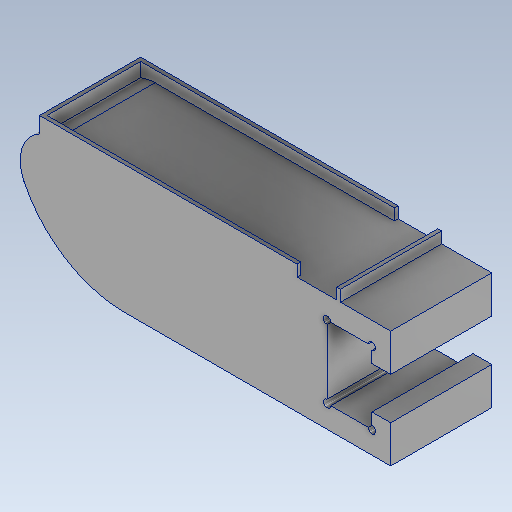
# Autodesk Inventor part: Finray_9_Kerbe_10deg_anschluss_erweitert_9_75 Nut
Saved by Autodesk Inventor 2025.2 (Build 292293000, 293)
## iProperties
Created: 2022-02-28
Part Number: Finray_9_Kerbe_10deg_anschluss_erweitert_9_75 Nut
Material: Generic
Document SubType Name: Modeling
Designer: richa
Density: 1 g/cm^3
Appearance: Aluminum - Flat
Author: richa
## iProperties of the stored document Maria_Greifer_3D-Druck.ipt
Created: 2024-11-10
Part Number: Maria_Greifer_3D-Druck
Material: Generisch
Document SubType Name: Modeling
Designer: maria
Density: 1 g/cm^3
Appearance: Vorgabe
Author: maria
Autodesk Inventor part; units mm, degrees
ref_plane "YZ Plane" through (0, 0, 0) normal (1, 0, 0) x (0, 1, 0)
ref_plane "XZ Plane" through (0, 0, 0) normal (0, 1, 0) x (-1, 0, 0)
ref_plane "XY Plane" through (0, 0, 0) normal (0, 0, 1) x (1, 0, 0)
sketch "Sketch5" plane through (0, 0, 0) normal (0, 0, 1) x (1, 0, 0)
  line L0 (50.5, -15.6) -> (50.5, -10.6)
  line L1 (50.5, -10.6) -> (48, -10.6)
  line L2 (48, -10.6) -> (48, -12.625)
  line L3 (42, -12.625) -> (42, -2.975)
  line L4 (48, -2.975) -> (48, -5)
  line L5 (48, -5) -> (50.5, -5)
  line L6 (50.5, -5) -> (50.5, 0)
  line L7 (50.5, 0) -> (5.8, 0)
  line L8 (42, -2.975) -> (48, -2.975)
  line L9 (42, -12.625) -> (48, -12.625)
  line L10 (50.5, -15.6) -> (5.8, -15.6)
  line L11 (5.8, -15.6) -> (0, -15.6)
  line L12 (0, -15.6) -> (0, 0)
  line L13 (0, 0) -> (7.8, 0)
  line L14 (40.5, 0) -> (40.5, -15.6)
  line L15 (39.5, -15.6) -> (39.5, 0)
  line L16 (0, -45.1294) -> (0, -34.3361)
  line L17 (0, -34.3361) -> (38.5, -34.3361)
  line L18 (38.5, -34.3361) -> (38.5, -45.1294)
  line L19 (38.5, -45.1294) -> (0, -45.1294)
  line L20 (38.5, -42.4105) -> (39.5, -42.4105)
  line L21 (39.5, -42.4105) -> (39.5, -38.1261)
  line L22 (39.5, -38.1261) -> (38.5, -38.1261)
  line L23 (39.5, -42.4105) -> (39.5, -49.5786)
  line L24 (39.5, -49.5786) -> (45, -49.5786)
  line L25 (45, -49.5786) -> (45, -34.3361)
  line L26 (45, -34.3361) -> (39.5, -34.3361)
  line L27 (39.5, -34.3361) -> (39.5, -38.1261)
  point P0 (7.8, 0)
  point P1 (39, -42.4105)
  dimension "d41" = 6
  dimension "d48" = 42
  dimension "d50" = 2.5
  dimension "d63" = 44.7
  dimension "d71" = 0
  dimension "d87" = 5.6
  dimension "d88" = 9.65
  dimension "d97" = 15.6
  dimension "d122" = 1.5
  dimension "d123" = 1
  dimension "d124" = 39.5
  dimension "d125" = 38.5
  dimension "d127" = 1
  dimension "d128" = 5.5
  constraints: 56 end point, 18 perpendicular, 8 point on line, 4 collinear, 3 horizontal, 3 parallel, 3 vertical, 1 midpoint
  measures "d41" distance between parallel lines of L2 L3
  measures "d48" distance from line of L3 L12.end
  measures "d50" distance of L4.end L5.end
  measures "d63" distance of L0.start L10.end
  measures "d71" distance from line of L12.end L7
  measures "d87" distance from line of L0.end L5
  measures "d88" distance of L3.start L3.end
  measures "d97" distance of L11.end L12.end
  measures "d122" distance between parallel lines of L3 L14
  measures "d123" distance between parallel lines of L14 L15
  measures "d124" distance between parallel lines of L12 L15
  measures "d125" distance of L18.end L16.start
  measures "d127" distance of L20.start L20.end
  measures "d128" distance of L23.end L24.end
extrude "Extrusion2" add sketch "Sketch5" along normal blind 13.5 contours L10 L14 L7 L6 L5 L4 L8 L3 L9 L2 L1 L0 | L10 L15 L7 L14 | L10 L11 L12 L13 L7 L15
fillet "Fillet2" radius 15 1 edges at (0, -15.6, 6.75)
sketch "Sketch11" plane through (0, 0, 13.5) normal (0, 0, 1) x (1, 0, 0)
  line L0 (42, -2.975) -> (48, -2.975) projected
  circle A0 centre (42, -2.975) radius 0.5
  line L1 (42, -12.625) -> (42, -2.975) projected
  circle A1 centre (42, -12.625) radius 0.5
  line L2 (48, -12.625) -> (42, -12.625) projected
  circle A2 centre (48, -12.625) radius 0.5
  line L3 (48, -2.975) -> (48, -5) projected
  circle A3 centre (48, -2.975) radius 0.5
  point P0 (0, 0)
  dimension "d99" = 1
  dimension "d100" = 1
  dimension "d101" = 1
  dimension "d102" = 1
  constraints: 4 centre point, 1 coincident
  measures "d99" diameter of A0
  measures "d100" diameter of A1
  measures "d101" diameter of A2
  measures "d102" diameter of A3
extrude "Extrusion7" cut sketch "Sketch11" against normal through all
fillet "Rundung3" radius 5 1 edges at (0, 0, 6.75)
sketch "Skizze17" plane through (50.5, 0, 13.5) normal (0, 1, 0) x (1, 0, 0)
  line L0 (-48.97, 13.5) -> (-35.5, 13.5) projected
  line L1 (-46.9, 0) -> (-46.4, 0)
  line L2 (-46.4, 0) -> (-46.4, 13.5)
  line L3 (-46.4, 13.5) -> (-46.9, 13.5)
  line L4 (-46.9, 13.5) -> (-46.9, 0)
  line L5 (-44.48, 0) -> (-49.48, 0) projected
  line L6 (-44.48, 0) -> (-44.48, 13.5) projected
  point P0 (-50.5, 13.5)
  point P1 (-48.97, 0)
  point P2 (-46.65, 0)
  dimension "d140" = 0.5
  dimension "d150" = 0
  dimension "d163" = 1.92
  constraints: 8 end point, 2 parallel, 1 horizontal, 1 midpoint, 1 perpendicular, 1 point on line
  measures "d140" distance between parallel lines of L2 L4
  measures "d150" distance from line of L5 point (-46.65, 0)
  measures "d163" distance between parallel lines of L2 L6
extrude "Extrusion12" add sketch "Skizze17" along normal mid plane 3 contours L0 L2 L1 L4
sketch "Skizze18" plane through (50.5, 0, 13.5) normal (0, 1, 0) x (1, 0, 0)
  line L0 (-6.6976, 0) -> (-6.6976, 13.5)
  line L1 (-46.4, 0) -> (-46.4, 13.5) projected
  line L2 (0, 13.5) -> (-44.48, 13.5) projected
  line L3 (0, 0) -> (-44.48, 0) projected
  line L4 (-7.1976, 0) -> (-7.1976, 13.5)
  line L5 (-7.1976, 13.5) -> (-6.6976, 13.5)
  line L6 (-7.1976, 0) -> (-6.6976, 0)
  point P0 (-50.5, 13.5)
  dimension "d160" = 0.5
  constraints: 8 end point, 2 point on line
  measures "d160" distance between parallel lines of L0 L4
extrude "Extrusion13" add sketch "Skizze18" along normal blind 1.5
sketch "Skizze19" plane through (6.02, 0, 13.5) normal (0, 1, 0) x (1, 0, 0)
  line L0 (44.48, 13.5) -> (0, 13.5) projected
  line L1 (-2.3517, 13) -> (37.6723, 13)
  line L2 (37.6723, 13) -> (37.6723, 13.5)
  line L3 (37.6723, 13.5) -> (-2.3517, 13.5)
  line L4 (-2.3517, 13.5) -> (-2.3517, 13)
  line L5 (-1.92, 0) -> (-1.92, 13.5) projected
  point P0 (-6.02, 13.5)
  point P1 (3.0824, 14.25)
  point P2 (16.6541, 14.25)
  point P3 (24.4324, 14.25)
  dimension "d159" = 0.5
  dimension "d162" = 0
  constraints: 8 end point, 1 horizontal, 1 parallel
  measures "d159" distance between parallel lines of L3 L1
  measures "d162" distance between parallel lines of L0 L3
extrude "Extrusion14" add sketch "Skizze19" along normal mid plane 3
sketch "Skizze20" plane through (6.02, 0, 13.5) normal (0, 1, 0) x (1, 0, 0)
  line L0 (36.7824, 14.5) -> (36.7824, 0) projected
  line L1 (-2.2337, 0) -> (36.7824, 0)
  line L2 (36.7824, 0) -> (36.7824, 0.5)
  line L3 (36.7824, 0.5) -> (-2.2337, 0.5)
  line L4 (-2.2337, 0.5) -> (-2.2337, 0)
  line L5 (37.2824, 0) -> (0, 0) projected
  point P0 (-6.02, 13.5)
  point P1 (36.7824, 14)
  dimension "d137" = 0
  dimension "d139" = 0.5
  constraints: 8 end point, 2 parallel, 1 horizontal, 1 perpendicular, 1 point on line
  measures "d137" distance between parallel lines of L1 L5
  measures "d139" distance between parallel lines of L1 L3
extrude "Extrusion15" add sketch "Skizze20" along normal mid plane 3
sketch "Skizze21" plane through (6.02, 0, 0.5) normal (0, 1, 0) x (1, 0, 0)
  line L0 (8.98, 0.5) -> (44.48, 0.5) projected
  line L1 (31.9824, 3.6397) -> (37.2824, 3.6397)
  line L2 (37.2824, 3.6397) -> (37.2824, -19.4506)
  line L3 (37.2824, -19.4506) -> (31.9824, -19.4506)
  line L4 (31.9824, -19.4506) -> (31.9824, 3.6397)
  line L5 (36.7824, 0) -> (36.7824, -13.5) projected
  line L6 (37.2824, 0) -> (37.2824, -13) projected
  point P0 (-6.02, 0.5)
  point P1 (37.2824, -0.5)
  dimension "d152" = 5.3
  dimension "d161" = 0
  constraints: 6 end point, 3 horizontal, 1 perpendicular, 4 other
  measures "d161" horizontal extent of L6
extrude "Extrusion16" cut sketch "Skizze21" along normal blind 3
equation "\"l1\" = 8"
body "Solid2"
